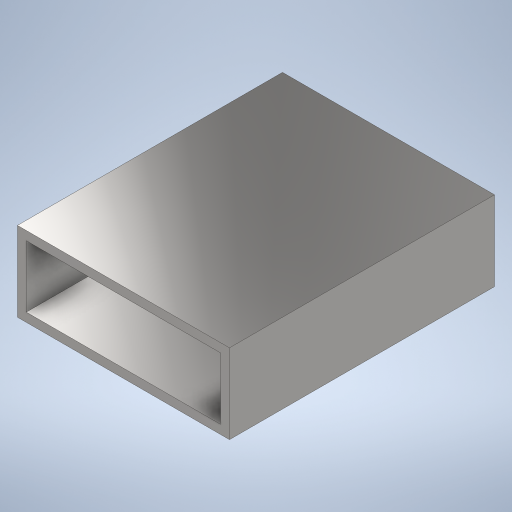
# Autodesk Inventor part: capa
Saved by Autodesk Inventor 2024.2 (Build 282272000, 272)
## iProperties
Created: 2024-04-15
Part Number: capa
Material: Steel, Alloy
Document SubType Name: Modeling
Designer: 082220022
Density: 7.73 g/cm^3
Appearance: Semi-Polished
Author: 082220022
Autodesk Inventor part; units mm, degrees
ref_plane "YZ Plane" through (0, 0, 0) normal (1, 0, 0) x (0, 1, 0)
ref_plane "XZ Plane" through (0, 0, 0) normal (0, 1, 0) x (-1, 0, 0)
ref_plane "XY Plane" through (0, 0, 0) normal (0, 0, 1) x (1, 0, 0)
sketch "Sketch1" plane through (0, 0, 0) normal (0, 0, 1) x (1, 0, 0)
  line L0 (-8.7146, 7.551) -> (3.2854, 7.551)
  line L1 (3.2854, 7.551) -> (3.2854, 3.051)
  line L2 (3.2854, 3.051) -> (-8.7146, 3.051)
  line L3 (-8.7146, 3.051) -> (-8.7146, 7.551)
  line L4 (2.7854, 7.051) -> (-8.2146, 7.051)
  line L5 (-8.2146, 7.051) -> (-8.2146, 3.551)
  line L6 (-8.2146, 3.551) -> (2.7854, 3.551)
  line L7 (2.7854, 3.551) -> (2.7854, 7.051)
  point P0 (0, 0)
  dimension "d0" = 12
  dimension "d1" = 4.5
  dimension "d2" = 0.5
  constraints: 16 end point, 4 parallel, 2 perpendicular, 1 horizontal, 3 other
  measures "d0" distance of L1.end L2.end
  measures "d1" distance of L0.end L1.end
  measures "d2" distance between parallel lines of L0 L4
extrude "Extrusion1" add sketch "Sketch1" along normal blind 15
body "Solid1"
